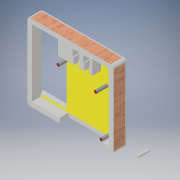
# Autodesk Inventor part: case_bottom_new
Saved by Autodesk Inventor 2017 (Build 210142000, 142)
## iProperties
Created: 2016-11-05
Part Number: case_bottom_new
Material: Generic
Document SubType Name: Modeling
Designer: radrajith
Density: 1 g/cm^3
Appearance: Default
Author: radrajith
Autodesk Inventor part; units mm, degrees
ref_plane "YZ Plane" through (0, 0, 0) normal (1, 0, 0) x (0, 1, 0)
ref_plane "XZ Plane" through (0, 0, 0) normal (0, 1, 0) x (-1, 0, 0)
ref_plane "XY Plane" through (0, 0, 0) normal (0, 0, 1) x (1, 0, 0)
sketch "Sketch1" plane through (0, 0, 0) normal (0, 0, 1) x (1, 0, 0)
  line L0 (-5, -5) -> (85, -5)
  line L1 (85, -5) -> (85, 75)
  line L2 (85, 75) -> (-5, 75)
  line L3 (-5, 75) -> (-5, -5)
  point P0 (0, 0)
  dimension "d0" = 90
  dimension "d1" = 80
  constraints: 8 end point, 2 parallel, 1 horizontal, 1 perpendicular
  measures "d0" distance of L2.end L1.end
  measures "d1" distance of L1.end L0.end
extrude "Extrusion1" add sketch "Sketch1" along normal blind 15
sketch "Sketch3" plane through (0, 0, 15) normal (0, 0, 1) x (1, 0, 0)
  line L0 (-0.1584, 0.1549) -> (79.8416, 0.1549)
  line L1 (79.8416, 0.1549) -> (79.8416, 70.1549)
  line L2 (79.8416, 70.1549) -> (-0.1584, 70.1549)
  line L3 (-0.1584, 70.1549) -> (-0.1584, 0.1549)
  point P0 (0, 0)
  dimension "d4" = 80
  dimension "d5" = 70
  constraints: 8 end point, 2 parallel, 1 horizontal, 1 perpendicular
  measures "d4" distance of L2.end L1.end
  measures "d5" distance of L1.end L0.end
extrude "Extrusion2" cut sketch "Sketch3" against normal blind 9
sketch "Sketch4" plane through (0, 0, 6) normal (0, 0, 1) x (1, 0, 0)
  circle A0 centre (75, 5) radius 1.55
  circle A1 centre (30, 50) radius 1.55
  circle A2 centre (68.99, 45) radius 1.55
  circle A3 centre (112.181, 7.869) radius 1.55
  point P0 (0, 0)
  dimension "d8" = 3.1
  dimension "d9" = 3.1
  dimension "d10" = 3.1
  dimension "d51" = 3.1
  constraints: 4 centre point
  measures "d8" diameter of A0
  measures "d9" diameter of A1
  measures "d10" diameter of A2
  measures "d51" diameter of A3
extrude "Extrusion3" add sketch "Sketch4" along normal blind 12
sketch "Sketch9" plane through (0, 0, 6) normal (0, 0, 1) x (1, 0, 0)
  line L0 (-0.1583, 67.5504) -> (26.8417, 67.5504)
  line L1 (26.8417, 67.5504) -> (26.8417, 2.5504)
  line L2 (26.8417, 2.5504) -> (-0.1583, 2.5504)
  line L3 (-0.1583, 2.5504) -> (-0.1583, 67.5504)
  point P0 (0, 0)
  dimension "d13" = 27
  dimension "d14" = 65
  constraints: 8 end point, 2 parallel, 1 horizontal, 1 perpendicular
  measures "d13" distance of L1.end L2.end
  measures "d14" distance of L0.end L1.end
extrude "Extrusion4" cut sketch "Sketch9" against normal blind 4
sketch "Sketch10" plane through (0, 0, 2) normal (0, 0, 1) x (1, 0, 0)
  line L0 (7, 64.5504) -> (20, 64.5504)
  line L1 (20, 64.5504) -> (20, 54.4354)
  line L2 (20, 54.4354) -> (7, 54.4354)
  line L3 (7, 54.4354) -> (7, 64.5504)
  line L4 (-0.1583, 67.5504) -> (26.8417, 67.5504) projected
  point P0 (0, 0)
  dimension "d54" = 3
  constraints: 8 end point, 2 parallel, 1 horizontal, 1 perpendicular
  measures "d54" distance between parallel lines of L0 L4
extrude "Extrusion5" cut sketch "Sketch10" against normal blind 3
sketch "Sketch12" plane through (-0.1584, 70.1549, 15) normal (0, -1, 0) x (1, 0, 0)
  line L0 (0, 0) -> (80, 0) projected
  line L1 (61.5, 0) -> (52.5, 0)
  line L2 (52.5, 0) -> (52.5, -9)
  line L3 (52.5, -9) -> (61.5, -9)
  line L4 (61.5, -9) -> (61.5, 0)
  line L5 (50.5, 0) -> (41.5, 0)
  line L6 (41.5, 0) -> (41.5, -9)
  line L7 (41.5, -9) -> (50.5, -9)
  line L8 (50.5, -9) -> (50.5, 0)
  point P0 (0.1584, -15)
  dimension "d44" = 9
  constraints: 16 end point, 4 parallel, 2 horizontal, 2 perpendicular
  measures "d44" distance between parallel lines of L8 L6
extrude "Extrusion7" add sketch "Sketch12" along normal blind 15
thread "Thread1" size "M3.5x0.6" class "6g" standard "ANSI Metric M Profile" full length
thread "Thread2" size "M3.5x0.6" class "6g" standard "ANSI Metric M Profile" full length
thread "Thread3" size "M3.5x0.6" class "6g" standard "ANSI Metric M Profile" full length
sketch "Sketch15" plane through (0, 0, 15) normal (0, 0, 1) x (1, 0, 0)
  line L0 (50.3416, 55.1549) -> (41.3416, 55.1549) projected
  line L1 (43.342, 55.1549) -> (48.342, 55.1549)
  line L2 (48.342, 55.1549) -> (48.342, 62.1549)
  line L3 (48.342, 62.1549) -> (43.342, 62.1549)
  line L4 (43.342, 62.1549) -> (43.342, 55.1549)
  point P0 (0, 0)
  dimension "d31" = 5
  dimension "d32" = 7
  constraints: 8 end point, 2 parallel, 1 horizontal, 1 perpendicular, 1 point on line
  measures "d31" distance of L3.end L2.end
  measures "d32" distance of L2.end L1.end
extrude "Extrusion9" cut sketch "Sketch15" against normal blind 9
sketch "Sketch16" plane through (0, 0, 15) normal (0, 0, 1) x (1, 0, 0)
  line L0 (61.3416, 55.1549) -> (52.3416, 55.1549) projected
  line L1 (54.342, 55.1549) -> (59.342, 55.1549)
  line L2 (59.342, 55.1549) -> (59.342, 62.1549)
  line L3 (59.342, 62.1549) -> (54.342, 62.1549)
  line L4 (54.342, 62.1549) -> (54.342, 55.1549)
  point P0 (0, 0)
  dimension "d35" = 5
  dimension "d36" = 7
  constraints: 8 end point, 2 parallel, 1 horizontal, 1 perpendicular, 1 point on line
  measures "d35" distance of L3.end L2.end
  measures "d36" distance of L2.end L1.end
extrude "Extrusion10" cut sketch "Sketch16" against normal blind 9
sketch "Sketch17" plane through (0, 0, 6) normal (0, 0, 1) x (1, 0, 0)
  line L0 (48.342, 55.1549) -> (48.342, 62.1549) projected
  line L1 (48.342, 62.1549) -> (43.342, 62.1549) projected
  line L2 (43.342, 62.1549) -> (43.342, 55.1549) projected
  line L3 (43.342, 55.1549) -> (41.3416, 55.1549) projected
  line L4 (41.3416, 55.1549) -> (41.3416, 70.1549) projected
  line L5 (41.3416, 70.1549) -> (-0.1584, 70.1549) projected
  line L6 (-0.1584, 70.1549) -> (-0.1584, 0.1549) projected
  line L7 (-0.1584, 0.1549) -> (79.8416, 0.1549) projected
  line L8 (79.8416, 0.1549) -> (79.8416, 70.1549) projected
  line L9 (79.8416, 70.1549) -> (61.3416, 70.1549) projected
  line L10 (61.3416, 70.1549) -> (61.3416, 55.1549) projected
  line L11 (61.3416, 55.1549) -> (59.342, 55.1549) projected
  line L12 (59.342, 55.1549) -> (59.342, 62.1549) projected
  line L13 (59.342, 62.1549) -> (54.342, 62.1549) projected
  line L14 (54.342, 62.1549) -> (54.342, 55.1549) projected
  line L15 (54.342, 55.1549) -> (52.3416, 55.1549) projected
  line L16 (52.3416, 55.1549) -> (52.3416, 70.1549) projected
  line L17 (52.3416, 70.1549) -> (50.3416, 70.1549) projected
  line L18 (50.3416, 70.1549) -> (50.3416, 55.1549) projected
  line L19 (50.3416, 55.1549) -> (48.342, 55.1549) projected
  line L20 (-0.1583, 67.5504) -> (-0.1583, 2.5504) projected
  line L21 (-0.1583, 2.5504) -> (26.8417, 2.5504) projected
  line L22 (26.8417, 2.5504) -> (26.8417, 67.5504) projected
  line L23 (26.8417, 67.5504) -> (-0.1583, 67.5504) projected
  circle A0 centre (30, 50) radius 1.55 projected
  circle A1 centre (75, 5) radius 1.55 projected
  circle A2 centre (68.99, 45) radius 1.55 projected
  line L24 (85, -5) -> (-5, -5) projected
  line L25 (-5, -5) -> (-5, 75) projected
  line L26 (-5, 75) -> (85, 75) projected
  line L27 (85, 75) -> (85, -5) projected
  line L28 (48.342, 55.1549) -> (48.342, 62.1549) projected
  line L29 (48.342, 62.1549) -> (43.342, 62.1549) projected
  line L30 (43.342, 62.1549) -> (43.342, 55.1549) projected
  line L31 (43.342, 55.1549) -> (41.3416, 55.1549) projected
  line L32 (41.3416, 55.1549) -> (41.3416, 70.1549) projected
  line L33 (41.3416, 70.1549) -> (-0.1584, 70.1549) projected
  line L34 (-0.1584, 70.1549) -> (-0.1584, 0.1549) projected
  line L35 (-0.1584, 0.1549) -> (79.8416, 0.1549) projected
  line L36 (79.8416, 0.1549) -> (79.8416, 70.1549) projected
  line L37 (79.8416, 70.1549) -> (61.3416, 70.1549) projected
  line L38 (61.3416, 70.1549) -> (61.3416, 55.1549) projected
  line L39 (61.3416, 55.1549) -> (59.342, 55.1549) projected
  line L40 (59.342, 55.1549) -> (59.342, 62.1549) projected
  line L41 (59.342, 62.1549) -> (54.342, 62.1549) projected
  line L42 (54.342, 62.1549) -> (54.342, 55.1549) projected
  line L43 (54.342, 55.1549) -> (52.3416, 55.1549) projected
  line L44 (52.3416, 55.1549) -> (52.3416, 70.1549) projected
  line L45 (52.3416, 70.1549) -> (50.3416, 70.1549) projected
  line L46 (50.3416, 70.1549) -> (50.3416, 55.1549) projected
  line L47 (50.3416, 55.1549) -> (48.342, 55.1549) projected
  circle A3 centre (30, 50) radius 1.55 projected
  circle A4 centre (75, 5) radius 1.55 projected
  circle A5 centre (68.99, 45) radius 1.55 projected
  line L48 (85, -5) -> (-5, -5) projected
  line L49 (-5, -5) -> (-5, 75) projected
  line L50 (-5, 75) -> (85, 75) projected
  line L51 (85, 75) -> (85, -5) projected
  line L52 (42.3418, 62.1549) -> (49.3418, 62.1549)
  line L53 (49.3418, 62.1549) -> (49.3418, 69.1549)
  line L54 (49.3418, 69.1549) -> (42.3418, 69.1549)
  line L55 (42.3418, 69.1549) -> (42.3418, 62.1549)
  line L56 (53.3418, 62.1549) -> (60.3418, 62.1549)
  line L57 (60.3418, 62.1549) -> (60.3418, 69.1549)
  line L58 (60.3418, 69.1549) -> (53.3418, 69.1549)
  line L59 (53.3418, 69.1549) -> (53.3418, 62.1549)
  line L60 (-0.1583, 67.5504) -> (-0.1583, 2.5504) projected
  line L61 (-0.1583, 2.5504) -> (26.8417, 2.5504) projected
  line L62 (26.8417, 2.5504) -> (26.8417, 67.5504) projected
  line L63 (26.8417, 67.5504) -> (-0.1583, 67.5504) projected
  circle A6 centre (112.181, 7.869) radius 1.55 projected
  circle A7 centre (112.181, 7.869) radius 1.55 projected
  point P0 (0, 0)
  dimension "d39" = 7
  dimension "d40" = 7
  dimension "d41" = 7
  constraints: 16 end point, 4 parallel, 2 horizontal, 2 perpendicular, 1 point on line
  measures "d39" distance of L53.end L52.end
  measures "d40" distance of L58.end L57.end
  measures "d41" distance of L57.end L56.end
extrude "Extrusion11" cut sketch "Sketch17" along normal blind 9 contours L1 L52 L55 L54 L53 | L56 L59 L58 L57 L13
sketch "Sketch18" plane through (50.3416, 70.1549, 15) normal (0, -1, 0) x (1, 0, 0)
  line L0 (0, 0) -> (2, 0)
  line L1 (2, 0) -> (2, -9)
  line L2 (2, -9) -> (0, -9)
  line L3 (0, -9) -> (0, 0)
  point P0 (-50.3416, -15)
  constraints: 8 end point, 2 parallel, 1 horizontal, 1 perpendicular
extrude "Extrusion12" add sketch "Sketch18" along normal blind 15
sketch "Sketch19" plane through (-0.1584, 70.1549, 6) normal (0, -1, 0) x (1, 0, 0)
  line L0 (41.5, 0) -> (41.5, 9) projected
  line L1 (0, 0) -> (41.5, 0) projected
  line L2 (41.5, 9) -> (40, 9)
  line L3 (40, 9) -> (40, 0)
  line L4 (40, 0) -> (41.5, 0)
  line L5 (41.5, 0) -> (41.5, 9)
  line L6 (61.5, 0) -> (80, 0) projected
  line L7 (61.5, 9) -> (63, 9)
  line L8 (63, 9) -> (63, 0)
  line L9 (63, 0) -> (61.5, 0)
  line L10 (61.5, 0) -> (61.5, 9)
  point P0 (0.1584, -6)
  dimension "d47" = 1.5
  dimension "d48" = 1.5
  constraints: 16 end point, 4 parallel, 2 horizontal, 2 perpendicular, 2 point on line
  measures "d47" distance of L4.end L3.end
  measures "d48" distance of L8.end L9.end
extrude "Extrusion13" add sketch "Sketch19" along normal blind 15
sketch "Sketch20" plane through (0, 0, 6) normal (0, 0, 1) x (1, 0, 0)
  point P0 (0, 0)
sketch "Sketch21" plane through (39.8416, 70.1549, 6) normal (-1, 0, 0) x (0, 0, 1)
  point P0 (-6, -70.1549)
sketch "Sketch22" plane through (0, 0, 6) normal (0, 0, 1) x (1, 0, 0)
  line L0 (43.342, 55.1549) -> (39.8416, 55.1549) projected
  line L1 (-0.1584, 70.1549) -> (39.8416, 70.1549) projected
  line L2 (39.8416, 55.1549) -> (27.066, 55.1549)
  line L3 (27.066, 55.1549) -> (27.066, 70.1549)
  line L4 (27.066, 70.1549) -> (39.8416, 70.1549)
  line L5 (39.8416, 70.1549) -> (39.8416, 55.1549)
  point P0 (0, 0)
  constraints: 8 end point, 2 parallel, 1 horizontal, 1 perpendicular, 1 point on line
extrude "Extrusion14" add sketch "Sketch22" along normal blind 9
fillet "Fillet1" radius 3 1 edges at (85, -5, 7.5)
fillet "Fillet2" radius 3 8 edges at (85, 75, 7.5) (-5, 75, 7.5) (-5, -5, 7.5) (-5, 35, 0) (40, 75, 0) (84.1213, -4.1213, 0) (38.5, -5, 0) (85, 36.5, 0)
sketch "Sketch23" plane through (-2, -5, 3) normal (0, -1, 0) x (1, 0, 0)
  line L0 (75.911, 12.0851) -> (30.911, 12.0851)
  line L1 (30.911, 12.0851) -> (30.911, 3.0851)
  line L2 (30.911, 3.0851) -> (75.911, 3.0851)
  line L3 (75.911, 3.0851) -> (75.911, 12.0851)
  point P0 (2, -3)
  dimension "d57" = 45
  dimension "d58" = 9
  constraints: 8 end point, 2 parallel, 1 horizontal, 1 perpendicular
  measures "d57" distance of L2.end L1.end
  measures "d58" distance between parallel lines of L0 L2
extrude "Extrusion15" cut sketch "Sketch23" against normal blind 6
fillet "Fillet3" radius 2 3 edges at (51.411, -5, 6.0851) (28.911, -5, 10.5426) (73.911, -5, 10.5426)
sketch "Sketch24" plane through (0, 0, 0) normal (0, 0, -1) x (-1, 0, 0)
  line L0 (-27, 1.5) -> (5, 1.5)
  line L1 (5, 1.5) -> (5, 68.5)
  line L2 (5, 68.5) -> (-27, 68.5)
  line L3 (-27, 68.5) -> (-27, 1.5)
  point P0 (0, 0)
  dimension "d62" = 32
  dimension "d63" = 67
  constraints: 8 end point, 2 parallel, 1 horizontal, 1 perpendicular
  measures "d62" distance of L2.end L1.end
  measures "d63" distance of L1.end L0.end
extrude "Extrusion16" cut sketch "Sketch24" against normal blind 5
sketch "Sketch25" plane through (0, 0, 0) normal (0, 0, -1) x (-1, 0, 0)
  line L0 (-27, 20) -> (-42, 20)
  line L1 (-42, 20) -> (-42, 50)
  line L2 (-42, 50) -> (-27, 50)
  line L3 (-27, 50) -> (-27, 20)
  point P0 (0, 0)
  dimension "d66" = 15
  dimension "d67" = 30
  constraints: 8 end point, 2 parallel, 1 horizontal, 1 perpendicular
  measures "d66" distance of L1.end L2.end
  measures "d67" distance of L0.end L1.end
extrude "Extrusion17" cut sketch "Sketch25" against normal blind 2
body "Solid1"
